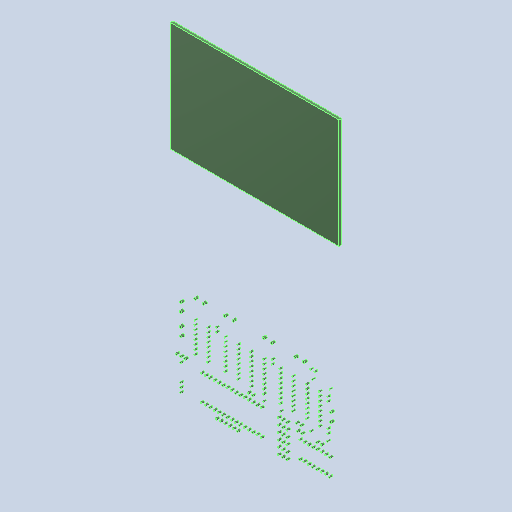
# Autodesk Inventor part: 璈_游_.kicad_pcb_Outline
Saved by Autodesk Inventor 2023.2 (Build 272271030, 271C)
## iProperties
Created: 2023-06-21
Part Number: 璈_游_.kicad_pcb_Outline
Material: Generic
Document SubType Name: Modeling
Designer: kao91
Density: 1 g/cm^3
Appearance: Board Outline
Author: kao91
Autodesk Inventor part; units mm, degrees
ref_plane "YZ Plane" through (0, 0, 0) normal (1, 0, 0) x (0, 1, 0)
ref_plane "XZ Plane" through (0, 0, 0) normal (0, 1, 0) x (-1, 0, 0)
ref_plane "XY Plane" through (0, 0, 0) normal (0, 0, 1) x (1, 0, 0)
sketch "Sketch1" plane through (0, 0, 0) normal (0, 0, 1) x (1, 0, 0)
  line L0 (36.4744, 32.2834) -> (136.3872, 32.2834)
  line L1 (136.3872, 32.2834) -> (136.3872, 97.2058)
  line L2 (136.3872, 97.2058) -> (36.4744, 97.2058)
  line L3 (36.4744, 97.2058) -> (36.4744, 32.2834)
  circle A0 centre (90.17, -73.67) radius 0.5
  circle A1 centre (87.63, -73.67) radius 0.5
  circle A2 centre (85.09, -73.67) radius 0.5
  circle A3 centre (82.55, -73.67) radius 0.5
  circle A4 centre (80.01, -73.67) radius 0.5
  circle A5 centre (77.47, -73.67) radius 0.5
  circle A6 centre (74.93, -73.67) radius 0.5
  circle A7 centre (72.39, -73.67) radius 0.5
  circle A8 centre (69.85, -73.67) radius 0.5
  circle A9 centre (67.31, -73.67) radius 0.5
  circle A10 centre (64.77, -73.67) radius 0.5
  circle A11 centre (62.23, -73.67) radius 0.5
  circle A12 centre (59.69, -73.67) radius 0.5
  circle A13 centre (57.15, -73.67) radius 0.5
  circle A14 centre (54.61, -73.67) radius 0.5
  circle A15 centre (54.61, -88.91) radius 0.5
  circle A16 centre (57.15, -88.91) radius 0.5
  circle A17 centre (59.69, -88.91) radius 0.5
  circle A18 centre (62.23, -88.91) radius 0.5
  circle A19 centre (64.77, -88.91) radius 0.5
  circle A20 centre (67.31, -88.91) radius 0.5
  circle A21 centre (69.85, -88.91) radius 0.5
  circle A22 centre (72.39, -88.91) radius 0.5
  circle A23 centre (74.93, -88.91) radius 0.5
  circle A24 centre (77.47, -88.91) radius 0.5
  circle A25 centre (80.01, -88.91) radius 0.5
  circle A26 centre (82.55, -88.91) radius 0.5
  circle A27 centre (85.09, -88.91) radius 0.5
  circle A28 centre (87.63, -88.91) radius 0.5
  circle A29 centre (90.17, -88.91) radius 0.5
  circle A30 centre (63.5, -45.76) radius 0.4
  circle A31 centre (63.5, -48.26) radius 0.4
  circle A32 centre (129.54, -48.26) radius 0.4
  circle A33 centre (129.54, -50.76) radius 0.4
  circle A34 centre (96.52, -45.72) radius 0.4
  circle A35 centre (96.52, -48.22) radius 0.4
  circle A36 centre (42.545, -86.995) radius 0.45
  circle A37 centre (42.545, -89.535) radius 0.45
  circle A38 centre (121.925, -39.37) radius 0.45
  circle A39 centre (119.385, -39.37) radius 0.45
  circle A40 centre (129.54, -67.31) radius 0.45
  circle A41 centre (129.54, -64.77) radius 0.45
  circle A42 centre (42.545, -55.88) radius 0.7
  circle A43 centre (42.545, -60.88) radius 0.7
  circle A44 centre (100.33, -81.28) radius 0.5
  circle A45 centre (102.87, -81.28) radius 0.5
  circle A46 centre (105.41, -81.28) radius 0.5
  circle A47 centre (100.33, -85.09) radius 0.5
  circle A48 centre (102.87, -85.09) radius 0.5
  circle A49 centre (105.41, -85.09) radius 0.5
  circle A50 centre (100.33, -88.9) radius 0.5
  circle A51 centre (102.87, -88.9) radius 0.5
  circle A52 centre (105.41, -88.9) radius 0.5
  circle A53 centre (100.33, -92.71) radius 0.5
  circle A54 centre (102.87, -92.71) radius 0.5
  circle A55 centre (105.41, -92.71) radius 0.5
  circle A56 centre (63.5, -92.71) radius 0.5
  circle A57 centre (66.04, -92.71) radius 0.5
  circle A58 centre (68.58, -92.71) radius 0.5
  circle A59 centre (71.12, -92.71) radius 0.5
  circle A60 centre (73.66, -92.71) radius 0.5
  circle A61 centre (76.2, -92.71) radius 0.5
  circle A62 centre (73.6854, -37.2364) radius 0.7
  circle A63 centre (68.6854, -37.2364) radius 0.7
  circle A64 centre (96.52, -37.2364) radius 0.7
  circle A65 centre (91.52, -37.2364) radius 0.7
  circle A66 centre (42.545, -43.22) radius 0.7
  circle A67 centre (42.545, -48.22) radius 0.7
  circle A68 centre (51.0771, -37.2832) radius 0.7
  circle A69 centre (56.0771, -37.2832) radius 0.7
  circle A70 centre (115.3376, -37.6174) radius 0.7
  circle A71 centre (110.3376, -37.6174) radius 0.7
  circle A72 centre (130.7084, -88.8492) radius 0.5
  circle A73 centre (128.1684, -88.8492) radius 0.5
  circle A74 centre (125.6284, -88.8492) radius 0.5
  circle A75 centre (123.0884, -88.8492) radius 0.5
  circle A76 centre (120.5484, -88.8492) radius 0.5
  circle A77 centre (118.0084, -88.8492) radius 0.5
  circle A78 centre (115.4684, -88.8492) radius 0.5
  circle A79 centre (112.9284, -88.8492) radius 0.5
  circle A80 centre (131.445, -60.325) radius 0.7
  circle A81 centre (131.445, -55.325) radius 0.7
  circle A82 centre (113.03, -78.74) radius 0.5
  circle A83 centre (115.57, -78.74) radius 0.5
  circle A84 centre (118.11, -78.74) radius 0.5
  circle A85 centre (120.65, -78.74) radius 0.5
  circle A86 centre (123.19, -78.74) radius 0.5
  circle A87 centre (125.73, -78.74) radius 0.5
  circle A88 centre (128.27, -78.74) radius 0.5
  circle A89 centre (130.81, -78.74) radius 0.5
  circle A90 centre (111.76, -74.93) radius 0.5
  circle A91 centre (114.3, -74.93) radius 0.5
  circle A92 centre (111.125, -71.12) radius 0.5
  circle A93 centre (113.665, -71.12) radius 0.5
  circle A94 centre (82.55, -69.85) radius 0.5
  circle A95 centre (85.09, -69.85) radius 0.5
  circle A96 centre (123.19, -74.93) radius 0.5
  circle A97 centre (125.73, -74.93) radius 0.5
  circle A98 centre (100.33, -73.66) radius 0.5
  circle A99 centre (102.87, -73.66) radius 0.5
  circle A100 centre (105.41, -73.66) radius 0.5
  circle A101 centre (100.33, -77.47) radius 0.5
  circle A102 centre (102.87, -77.47) radius 0.5
  circle A103 centre (105.41, -77.47) radius 0.5
  circle A104 centre (101.6, -69.85) radius 0.4
  circle A105 centre (91.44, -69.85) radius 0.4
  circle A106 centre (42.545, -84.455) radius 0.4
  circle A107 centre (42.545, -74.295) radius 0.4
  circle A108 centre (120.65, -43.815) radius 0.4
  circle A109 centre (130.81, -43.815) radius 0.4
  circle A110 centre (129.54, -71.12) radius 0.4
  circle A111 centre (119.38, -71.12) radius 0.4
  circle A112 centre (40.005, -71.12) radius 0.55
  circle A113 centre (42.545, -71.12) radius 0.55
  circle A114 centre (45.085, -71.12) radius 0.55
  circle A115 centre (68.58, -48.26) radius 0.4
  circle A116 centre (68.58, -50.8) radius 0.4
  circle A117 centre (68.58, -53.34) radius 0.4
  circle A118 centre (68.58, -55.88) radius 0.4
  circle A119 centre (68.58, -58.42) radius 0.4
  circle A120 centre (68.58, -60.96) radius 0.4
  circle A121 centre (68.58, -63.5) radius 0.4
  circle A122 centre (68.58, -66.04) radius 0.4
  circle A123 centre (76.2, -66.04) radius 0.4
  circle A124 centre (76.2, -63.5) radius 0.4
  circle A125 centre (76.2, -60.96) radius 0.4
  circle A126 centre (76.2, -58.42) radius 0.4
  circle A127 centre (76.2, -55.88) radius 0.4
  circle A128 centre (76.2, -53.34) radius 0.4
  circle A129 centre (76.2, -50.8) radius 0.4
  circle A130 centre (76.2, -48.26) radius 0.4
  circle A131 centre (108.8, -66.04) radius 0.4
  circle A132 centre (108.8, -63.5) radius 0.4
  circle A133 centre (108.8, -60.96) radius 0.4
  circle A134 centre (108.8, -58.42) radius 0.4
  circle A135 centre (108.8, -55.88) radius 0.4
  circle A136 centre (108.8, -53.34) radius 0.4
  circle A137 centre (108.8, -50.8) radius 0.4
  circle A138 centre (108.8, -48.26) radius 0.4
  circle A139 centre (101.18, -48.26) radius 0.4
  circle A140 centre (101.18, -50.8) radius 0.4
  circle A141 centre (101.18, -53.34) radius 0.4
  circle A142 centre (101.18, -55.88) radius 0.4
  circle A143 centre (101.18, -58.42) radius 0.4
  circle A144 centre (101.18, -60.96) radius 0.4
  circle A145 centre (101.18, -63.5) radius 0.4
  circle A146 centre (101.18, -66.04) radius 0.4
  circle A147 centre (50.8, -48.4124) radius 0.4
  circle A148 centre (50.8, -50.9524) radius 0.4
  circle A149 centre (50.8, -53.4924) radius 0.4
  circle A150 centre (50.8, -56.0324) radius 0.4
  circle A151 centre (50.8, -58.5724) radius 0.4
  circle A152 centre (50.8, -61.1124) radius 0.4
  circle A153 centre (50.8, -63.6524) radius 0.4
  circle A154 centre (50.8, -66.1924) radius 0.4
  circle A155 centre (58.42, -66.1924) radius 0.4
  circle A156 centre (58.42, -63.6524) radius 0.4
  circle A157 centre (58.42, -61.1124) radius 0.4
  circle A158 centre (58.42, -58.5724) radius 0.4
  circle A159 centre (58.42, -56.0324) radius 0.4
  circle A160 centre (58.42, -53.4924) radius 0.4
  circle A161 centre (58.42, -50.9524) radius 0.4
  circle A162 centre (58.42, -48.4124) radius 0.4
  circle A163 centre (83.82, -48.26) radius 0.4
  circle A164 centre (83.82, -50.8) radius 0.4
  circle A165 centre (83.82, -53.34) radius 0.4
  circle A166 centre (83.82, -55.88) radius 0.4
  circle A167 centre (83.82, -58.42) radius 0.4
  circle A168 centre (83.82, -60.96) radius 0.4
  circle A169 centre (83.82, -63.5) radius 0.4
  circle A170 centre (83.82, -66.04) radius 0.4
  circle A171 centre (91.44, -66.04) radius 0.4
  circle A172 centre (91.44, -63.5) radius 0.4
  circle A173 centre (91.44, -60.96) radius 0.4
  circle A174 centre (91.44, -58.42) radius 0.4
  circle A175 centre (91.44, -55.88) radius 0.4
  circle A176 centre (91.44, -53.34) radius 0.4
  circle A177 centre (91.44, -50.8) radius 0.4
  circle A178 centre (91.44, -48.26) radius 0.4
  circle A179 centre (116.84, -48.26) radius 0.4
  circle A180 centre (116.84, -50.8) radius 0.4
  circle A181 centre (116.84, -53.34) radius 0.4
  circle A182 centre (116.84, -55.88) radius 0.4
  circle A183 centre (116.84, -58.42) radius 0.4
  circle A184 centre (116.84, -60.96) radius 0.4
  circle A185 centre (116.84, -63.5) radius 0.4
  circle A186 centre (116.84, -66.04) radius 0.4
  circle A187 centre (124.46, -66.04) radius 0.4
  circle A188 centre (124.46, -63.5) radius 0.4
  circle A189 centre (124.46, -60.96) radius 0.4
  circle A190 centre (124.46, -58.42) radius 0.4
  circle A191 centre (124.46, -55.88) radius 0.4
  circle A192 centre (124.46, -53.34) radius 0.4
  circle A193 centre (124.46, -50.8) radius 0.4
  circle A194 centre (124.46, -48.26) radius 0.4
  constraints: 195 centre point, 8 end point
extrude "璈_游_.kicad_pcb_Outline" add sketch "Sketch1" along normal blind 1.6
body "Solid1"
